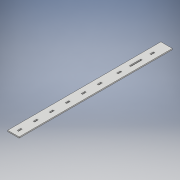
# Autodesk Inventor part: poprz_teownik
Saved by Autodesk Inventor 2017 (Build 210142000, 142)
## iProperties
Created: 2019-10-28
Part Number: poprz_teownik
Material: Ogólny
Document SubType Name: Modeling
Designer: patry
Density: 1 g/cm^3
Appearance: Domyślna
Author: patry
Autodesk Inventor part; units mm, degrees
ref_plane "YZ Plane" through (0, 0, 0) normal (1, 0, 0) x (0, 1, 0)
ref_plane "XZ Plane" through (0, 0, 0) normal (0, 1, 0) x (-1, 0, 0)
ref_plane "XY Plane" through (0, 0, 0) normal (0, 0, 1) x (1, 0, 0)
sketch "Szkic1" plane through (0, 0, 0) normal (0, 0, 1) x (1, 0, 0)
  line L0 (-36.75, 55) -> (13.25, 55)
  line L1 (13.25, 55) -> (13.25, -615)
  line L2 (13.25, -615) -> (-36.75, -615)
  line L3 (-36.75, -615) -> (-36.75, 55)
  line L4 (-15, -579) -> (-9, -579)
  line L5 (-9, -579) -> (-9, -595)
  line L6 (-9, -595) -> (-15, -595)
  line L7 (-15, -595) -> (-15, -579)
  line L8 (-15, -509) -> (-9, -509)
  line L9 (-9, -509) -> (-9, -525)
  line L10 (-9, -525) -> (-15, -525)
  line L11 (-15, -525) -> (-15, -509)
  line L12 (-15, -439) -> (-9, -439)
  line L13 (-9, -439) -> (-9, -455)
  line L14 (-9, -455) -> (-15, -455)
  line L15 (-15, -455) -> (-15, -439)
  line L16 (-15, -369) -> (-9, -369)
  line L17 (-9, -369) -> (-9, -385)
  line L18 (-9, -385) -> (-15, -385)
  line L19 (-15, -385) -> (-15, -369)
  line L20 (-15, -299) -> (-9, -299)
  line L21 (-9, -299) -> (-9, -315)
  line L22 (-9, -315) -> (-15, -315)
  line L23 (-15, -315) -> (-15, -299)
  line L24 (-15, -229) -> (-9, -229)
  line L25 (-9, -229) -> (-9, -245)
  line L26 (-9, -245) -> (-15, -245)
  line L27 (-15, -245) -> (-15, -229)
  line L28 (-15, -144) -> (-9, -144)
  line L29 (-9, -144) -> (-9, -160)
  line L30 (-9, -160) -> (-15, -160)
  line L31 (-15, -160) -> (-15, -144)
  line L32 (-15, -54) -> (-9, -54)
  line L33 (-9, -54) -> (-9, -105)
  line L34 (-9, -105) -> (-15, -105)
  line L35 (-15, -105) -> (-15, -54)
  line L36 (-9, -15) -> (-15, -15)
  line L37 (-15, -15) -> (-15, 1)
  line L38 (-15, 1) -> (-9, 1)
  line L39 (-9, 1) -> (-9, -15)
  point P0 (0, 0)
  point P1 (-9, -152)
  point P2 (-9, -7)
  point P3 (-9, -79.5)
  dimension "d0" = 50
  dimension "d1" = 670
  dimension "d2" = 6
  dimension "d3" = 16
  dimension "d4" = 22.25
  dimension "d5" = 20
  dimension "d8" = 70
  dimension "d13" = 16
  dimension "d14" = 6
  dimension "d16" = 69
  dimension "d20" = 6
  dimension "d21" = 51
  dimension "d26" = 39
  dimension "d27" = 6
  dimension "d28" = 16
  dimension "d29" = 39
  constraints: 80 end point, 9 parallel, 7 perpendicular, 4 horizontal, 3 midpoint, 2 vertical alignment, 1 vertical, 40 other
  measures "d0" distance of L1.end L2.end
  measures "d1" distance of L0.end L1.end
  measures "d2" distance of L5.end L6.end
  measures "d3" distance of L4.end L5.end
  measures "d4" distance between parallel lines of L1 L5
  measures "d5" distance between parallel lines of L2 L6
  measures "d8" distance of L4.start L8.start
  measures "d13" distance of L28.end L30.start
  measures "d14" distance of L28.start L28.end
  measures "d16" distance from line of L24 L30.end
  measures "d20" distance of L33.end L34.end
  measures "d21" distance of L32.end L33.end
  measures "d26" distance between parallel lines of L34 L28
  measures "d27" distance of L37.end L38.end
  measures "d28" distance of L36.end L37.end
  measures "d29" distance between parallel lines of L32 L36
extrude "Wyciągnięcie proste1" add sketch "Szkic1" along normal blind 5
equation "\"d29\" = d26"
